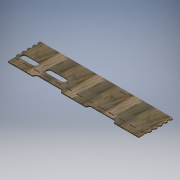
# Autodesk Inventor part: Dietro
Saved by Autodesk Inventor 2018.3 (Build 223284000, 284)
## iProperties
Created: 2019-03-05
Part Number: Dietro
Material: Generico
Document SubType Name: Modeling
Designer: AlfyPc
Density: 1 g/cm^3
Appearance: Legno alla deriva
Author: AlfyPc
Autodesk Inventor part; units mm, degrees
(part 1 of 5)
ref_plane "YZ Plane" through (0, 0, 0) normal (1, 0, 0) x (0, 1, 0)
ref_plane "XZ Plane" through (0, 0, 0) normal (0, 1, 0) x (-1, 0, 0)
ref_plane "XY Plane" through (0, 0, 0) normal (0, 0, 1) x (1, 0, 0)
sketch "Schizzo1" plane through (0, 0, 0) normal (0, 0, 1) x (1, 0, 0)
  line L0 (-15, -4) -> (-15, 0) construction
  line L1 (-34, 0) -> (-15, 0) construction
  line L2 (-53, 0) -> (-34, 0) construction
  line L3 (-72, 0) -> (-53, 0) construction
  line L4 (-91, 0) -> (-72, 0) construction
  line L5 (-110, 0) -> (-91, 0) construction
  line L6 (-129, 0) -> (-110, 0) construction
  line L7 (-148, 0) -> (-129, 0) construction
  line L8 (-167, 0) -> (-148, 0) construction
  line L9 (-186, 0) -> (-167, 0) construction
  line L10 (-205, 0) -> (-186, 0) construction
  line L11 (-224, 0) -> (-205, 0) construction
  line L12 (-243, 0) -> (-224, 0) construction
  line L13 (-262, 0) -> (-243, 0) construction
  line L14 (-281, 0) -> (-262, 0) construction
  line L15 (-300, 0) -> (-281, 0) construction
  line L16 (-319, 0) -> (-300, 0) construction
  line L17 (-338, 0) -> (-319, 0) construction
  line L18 (-357, 0) -> (-338, 0) construction
  line L19 (-376, 0) -> (-357, 0) construction
  line L20 (-395, 0) -> (-376, 0) construction
  line L21 (-414, 0) -> (-395, 0) construction
  line L22 (-433, 0) -> (-414, 0) construction
  line L23 (-452, 0) -> (-433, 0) construction
  line L24 (-471, 0) -> (-452, 0) construction
  line L25 (-471, -4) -> (-471, 0) construction
  line L26 (-452, -4) -> (-471, -4) construction
  line L27 (-452, 0) -> (-452, -4) construction
  line L28 (-15, -4) -> (-34, -4) construction
  line L29 (4, -4) -> (-15, -4) construction
  line L30 (4, 0) -> (4, -4) construction
  line L31 (-15, 0) -> (4, 0) construction
  line L32 (-34, 0) -> (-34, -4) construction
  line L33 (-53, -4) -> (-53, 0) construction
  line L34 (-34, -4) -> (-53, -4) construction
  line L35 (-72, 0) -> (-72, -4) construction
  line L36 (-53, -4) -> (-72, -4) construction
  line L37 (-91, -4) -> (-91, 0) construction
  line L38 (-72, -4) -> (-91, -4) construction
  line L39 (-110, 0) -> (-110, -4) construction
  line L40 (-91, -4) -> (-110, -4) construction
  line L41 (-129, -4) -> (-129, 0) construction
  line L42 (-110, -4) -> (-129, -4) construction
  line L43 (-148, 0) -> (-148, -4) construction
  line L44 (-129, -4) -> (-148, -4) construction
  line L45 (-167, -4) -> (-167, 0) construction
  line L46 (-148, -4) -> (-167, -4) construction
  line L47 (-186, 0) -> (-186, -4) construction
  line L48 (-167, -4) -> (-186, -4) construction
  line L49 (-205, -4) -> (-205, 0) construction
  line L50 (-186, -4) -> (-205, -4) construction
  line L51 (-224, 0) -> (-224, -4) construction
  line L52 (-205, -4) -> (-224, -4) construction
  line L53 (-243, -4) -> (-243, 0) construction
  line L54 (-224, -4) -> (-243, -4) construction
  line L55 (-262, 0) -> (-262, -4) construction
  line L56 (-243, -4) -> (-262, -4) construction
  line L57 (-281, -4) -> (-281, 0) construction
  line L58 (-262, -4) -> (-281, -4) construction
  line L59 (-300, 0) -> (-300, -4) construction
  line L60 (-281, -4) -> (-300, -4) construction
  line L61 (-319, -4) -> (-319, 0) construction
  line L62 (-300, -4) -> (-319, -4) construction
  line L63 (-338, 0) -> (-338, -4) construction
  line L64 (-319, -4) -> (-338, -4) construction
  line L65 (-357, -4) -> (-357, 0) construction
  line L66 (-338, -4) -> (-357, -4) construction
  line L67 (-376, 0) -> (-376, -4) construction
  line L68 (-357, -4) -> (-376, -4) construction
  line L69 (-395, -4) -> (-395, 0) construction
  line L70 (-376, -4) -> (-395, -4) construction
  line L71 (-414, 0) -> (-414, -4) construction
  line L72 (-395, -4) -> (-414, -4) construction
  line L73 (-433, -4) -> (-433, 0) construction
  line L74 (-414, -4) -> (-433, -4) construction
  line L75 (-433, -4) -> (-452, -4) construction
  line L76 (4, 95) -> (4, 0) construction
  line L77 (4, 0) -> (0, 0) construction
  line L78 (0, 0) -> (0, 95) construction
  line L79 (0, 95) -> (4, 95) construction
  line L80 (4, -4) -> (4, -24) construction
  line L81 (4, -24) -> (0, -24) construction
  line L82 (0, -24) -> (0, -4) construction
  line L83 (0, -4) -> (4, -4) construction
  line L84 (-381, -24) -> (-471, -24)
  line L85 (-471, -24) -> (-471, 95)
  line L86 (-471, 95) -> (4, 95)
  line L87 (4, 95) -> (4, -24)
  line L88 (-376, -19) -> (-376, -19)
  line L89 (-371, -14) -> (-286, -14)
  line L90 (-281, -19) -> (-281, -19)
  line L91 (-276, -24) -> (-191, -24)
  arc A0 (-381, -24) -> (-376, -19) centre (-381, -19) ccw
  arc A1 (-371, -14) -> (-376, -19) centre (-371, -19) ccw
  arc A2 (-281, -19) -> (-286, -14) centre (-286, -19) ccw
  arc A3 (-281, -19) -> (-276, -24) centre (-276, -19) ccw
  line L92 (-186, -19) -> (-186, -19)
  line L93 (-181, -14) -> (-96, -14)
  line L94 (-91, -19) -> (-91, -19)
  line L95 (-86, -24) -> (4, -24)
  arc A4 (-191, -24) -> (-186, -19) centre (-191, -19) ccw
  arc A5 (-181, -14) -> (-186, -19) centre (-181, -19) ccw
  arc A6 (-91, -19) -> (-96, -14) centre (-96, -19) ccw
  arc A7 (-91, -19) -> (-86, -24) centre (-86, -19) ccw
  line L96 (-15, -4) -> (4, -4) projected
  line L97 (4, 0) -> (4, -4) projected
  line L98 (4, 0) -> (-15, 0) projected
  line L99 (-15, 0) -> (-15, -4) projected
  line L100 (-53, -4) -> (-34, -4) projected
  line L101 (-34, 0) -> (-34, -4) projected
  line L102 (-53, 0) -> (-34, 0) projected
  line L103 (-53, 0) -> (-53, -4) projected
  line L104 (-91, -4) -> (-72, -4) projected
  line L105 (-72, 0) -> (-72, -4) projected
  line L106 (-91, 0) -> (-72, 0) projected
  line L107 (-91, 0) -> (-91, -4) projected
  line L108 (-129, -4) -> (-110, -4) projected
  line L109 (-110, 0) -> (-110, -4) projected
  line L110 (-129, 0) -> (-110, 0) projected
  line L111 (-129, 0) -> (-129, -4) projected
  line L112 (-167, -4) -> (-148, -4) projected
  line L113 (-148, 0) -> (-148, -4) projected
  line L114 (-167, 0) -> (-148, 0) projected
  line L115 (-167, 0) -> (-167, -4) projected
  line L116 (-205, -4) -> (-186, -4) projected
  line L117 (-186, 0) -> (-186, -4) projected
  line L118 (-205, 0) -> (-186, 0) projected
  line L119 (-205, 0) -> (-205, -4) projected
  line L120 (-243, -4) -> (-224, -4) projected
  line L121 (-224, 0) -> (-224, -4) projected
  line L122 (-243, 0) -> (-224, 0) projected
  line L123 (-243, 0) -> (-243, -4) projected
  line L124 (-281, -4) -> (-262, -4) projected
  line L125 (-262, 0) -> (-262, -4) projected
  line L126 (-281, 0) -> (-262, 0) projected
  line L127 (-281, 0) -> (-281, -4) projected
  line L128 (-319, -4) -> (-300, -4) projected
  line L129 (-300, 0) -> (-300, -4) projected
  line L130 (-319, 0) -> (-300, 0) projected
  line L131 (-319, 0) -> (-319, -4) projected
  line L132 (-357, -4) -> (-338, -4) projected
  line L133 (-338, 0) -> (-338, -4) projected
  line L134 (-357, 0) -> (-338, 0) projected
  line L135 (-357, 0) -> (-357, -4) projected
  line L136 (-395, -4) -> (-376, -4) projected
  line L137 (-376, 0) -> (-376, -4) projected
  line L138 (-395, 0) -> (-376, 0) projected
  line L139 (-395, 0) -> (-395, -4) projected
  line L140 (-433, -4) -> (-414, -4) projected
  line L141 (-414, 0) -> (-414, -4) projected
  line L142 (-433, 0) -> (-414, 0) projected
  line L143 (-433, 0) -> (-433, -4) projected
  line L144 (-471, -4) -> (-452, -4) projected
  line L145 (-452, 0) -> (-452, -4) projected
  line L146 (-471, 0) -> (-452, 0) projected
  line L147 (-471, 0) -> (-471, -4) projected
  line L148 (-361.5, 18) -> (-309.6633, 18) construction
  line L149 (-361.5, 8.6924) -> (-309.6633, 8.6924)
  line L150 (-309.6633, 27.3076) -> (-361.5, 27.3076)
  arc A8 (-361.5, 27.3076) -> (-361.5, 8.6924) centre (-361.5, 18) ccw
  arc A9 (-309.6633, 8.6924) -> (-309.6633, 27.3076) centre (-309.6633, 18) ccw
  line L151 (-451.5, 18) -> (-411.5, 18) construction
  line L152 (-451.5, 28) -> (-411.5, 28)
  line L153 (-411.5, 8) -> (-451.5, 8)
  arc A10 (-451.5, 28) -> (-451.5, 8) centre (-451.5, 18) ccw
  arc A11 (-411.5, 8) -> (-411.5, 28) centre (-411.5, 18) ccw
  point P0 (-376, -14)
  point P1 (-281, -14)
  point P2 (-281, -24)
  point P3 (-186, -24)
  point P4 (-186, -14)
  point P5 (-91, -14)
  point P6 (-335.5816, 18)
  point P7 (-431.5, 18)
  dimension "d2" = 95
  dimension "d3" = 90
  dimension "d4" = 95
  dimension "d5" = 5
  dimension "d6" = 90
  dimension "d7" = 95
  dimension "d8" = 5
  dimension "d22" = 40
  dimension "d23" = 18
  dimension "d24" = 20
  dimension "d25" = 50
  constraints: 208 end point, 56 horizontal, 31 vertical, 24 point on circle, 24 tangent, 17 point on line, 12 centre point, 6 equal radius, 6 perpendicular, 4 parallel, 2 midpoint, 57 other
  measures "d2" distance of point (-376, -14) point (-281, -14)
  measures "d3" angle of L88 L89
  measures "d4" distance of point (-281, -24) point (-186, -24)
  measures "d5" radius of A0
  measures "d6" distance of L84.start L84.end
  measures "d7" distance of point (-186, -14) point (-91, -14)
  measures "d8" radius of A4
  measures "d22" distance of L151.start L151.end
  measures "d23" distance between parallel lines of L22 L151
  measures "d24" distance between parallel lines of L153 L152
  measures "d25" distance of L151.end L148.start
extrude "Estrusione1" add sketch "Schizzo1" along normal blind 4 contours L84 L85 L144 L145 L146 L86 L87 L98 L99 L96 L95 A7 A6 L93 A5 A4 L91 A3 A2 L89 A1 A0
sketch "Schizzo2" plane through (0, 0, 4) normal (0, 0, 1) x (1, 0, 0)
  line L0 (0, -4) -> (0, -24) projected
  line L1 (0, -24) -> (4, -24) projected
  line L2 (4, -4) -> (4, -24) projected
  line L3 (0, -4) -> (4, -4) projected
  line L4 (0, -4) -> (0, -24) construction
  line L5 (4, -4) -> (4, -24) construction
  line L6 (-467, -4) -> (-471, -4) projected
  line L7 (-471, -24) -> (-471, -4) projected
  line L8 (-467, -24) -> (-471, -24) projected
  line L9 (-467, -24) -> (-467, -4) projected
  line L10 (-467, 0) -> (-467, 9.5) construction
  line L11 (-471, 0) -> (-471, 9.5) construction
  line L12 (4, 0) -> (4, 95) projected
  line L13 (0, 0) -> (4, 0)
  line L14 (4, 0) -> (4, 9.5)
  line L15 (4, 9.5) -> (0, 9.5)
  line L16 (0, 9.5) -> (0, 0)
  line L17 (-471, 95) -> (-471, 0) projected
  line L18 (-467, 0) -> (-471, 0)
  line L19 (-471, 0) -> (-471, 9.5)
  line L20 (-471, 9.5) -> (-467, 9.5)
  line L21 (-467, 9.5) -> (-467, 0)
  line L22 (0, 19) -> (0, 9.5)
  line L23 (0, 9.5) -> (4, 9.5)
  line L24 (4, 9.5) -> (4, 19)
  line L25 (4, 19) -> (0, 19)
  line L26 (-467, 19) -> (-467, 9.5)
  line L27 (-467, 9.5) -> (-471, 9.5)
  line L28 (-471, 9.5) -> (-471, 19)
  line L29 (-471, 19) -> (-467, 19)
  line L30 (0, 28.5) -> (0, 19)
  line L31 (0, 19) -> (4, 19)
  line L32 (4, 19) -> (4, 28.5)
  line L33 (4, 28.5) -> (0, 28.5)
  line L34 (-467, 28.5) -> (-467, 19)
  line L35 (-467, 19) -> (-471, 19)
  line L36 (-471, 19) -> (-471, 28.5)
  line L37 (-471, 28.5) -> (-467, 28.5)
  line L38 (0, 38) -> (0, 28.5)
  line L39 (0, 28.5) -> (4, 28.5)
  line L40 (4, 28.5) -> (4, 38)
  line L41 (4, 38) -> (0, 38)
  line L42 (-467, 38) -> (-467, 28.5)
  line L43 (-467, 28.5) -> (-471, 28.5)
  line L44 (-471, 28.5) -> (-471, 38)
  line L45 (-471, 38) -> (-467, 38)
  line L46 (0, 47.5) -> (0, 38)
  line L47 (0, 38) -> (4, 38)
  line L48 (4, 38) -> (4, 47.5)
  line L49 (4, 47.5) -> (0, 47.5)
  line L50 (-467, 47.5) -> (-467, 38)
  line L51 (-467, 38) -> (-471, 38)
  line L52 (-471, 38) -> (-471, 47.5)
  line L53 (-471, 47.5) -> (-467, 47.5)
  line L54 (0, 57) -> (0, 47.5)
  line L55 (0, 47.5) -> (4, 47.5)
  line L56 (4, 47.5) -> (4, 57)
  line L57 (4, 57) -> (0, 57)
  line L58 (-467, 57) -> (-467, 47.5)
  line L59 (-467, 47.5) -> (-471, 47.5)
  line L60 (-471, 47.5) -> (-471, 57)
  line L61 (-471, 57) -> (-467, 57)
  line L62 (0, 66.5) -> (0, 57)
  line L63 (0, 57) -> (4, 57)
  line L64 (4, 57) -> (4, 66.5)
  line L65 (4, 66.5) -> (0, 66.5)
  line L66 (-467, 66.5) -> (-467, 57)
  line L67 (-467, 57) -> (-471, 57)
  line L68 (-471, 57) -> (-471, 66.5)
  line L69 (-471, 66.5) -> (-467, 66.5)
  line L70 (0, 76) -> (0, 66.5)
  line L71 (0, 66.5) -> (4, 66.5)
  line L72 (4, 66.5) -> (4, 76)
  line L73 (4, 76) -> (0, 76)
  line L74 (-467, 76) -> (-467, 66.5)
  line L75 (-467, 66.5) -> (-471, 66.5)
  line L76 (-471, 66.5) -> (-471, 76)
  line L77 (-471, 76) -> (-467, 76)
  line L78 (0, 85.5) -> (0, 76)
  line L79 (0, 76) -> (4, 76)
  line L80 (4, 76) -> (4, 85.5)
  line L81 (4, 85.5) -> (0, 85.5)
  line L82 (-467, 85.5) -> (-467, 76)
  line L83 (-467, 76) -> (-471, 76)
  line L84 (-471, 76) -> (-471, 85.5)
  line L85 (-471, 85.5) -> (-467, 85.5)
  line L86 (0, 95) -> (0, 85.5)
  line L87 (0, 85.5) -> (4, 85.5)
  line L88 (4, 85.5) -> (4, 95)
  line L89 (4, 95) -> (0, 95)
  line L90 (-467, 95) -> (-467, 85.5)
  line L91 (-467, 85.5) -> (-471, 85.5)
  line L92 (-471, 85.5) -> (-471, 95)
  line L93 (-471, 95) -> (-467, 95)
  line L94 (0, -24) -> (4, -24) projected
  line L95 (0, -4) -> (4, -4) projected
  line L96 (-467, 9.5) -> (-471, 9.5) projected
  line L97 (-471, 0) -> (-467, 0) projected
  point P0 (4, 9.5)
  point P1 (-471, 9.5)
  point P2 (4, 19)
  point P3 (-471, 19)
  point P4 (4, 28.5)
  point P5 (-471, 28.5)
  point P6 (4, 38)
  point P7 (-471, 38)
  point P8 (4, 47.5)
  point P9 (-471, 47.5)
  point P10 (4, 57)
  point P11 (-471, 57)
  point P12 (4, 66.5)
  point P13 (-471, 66.5)
  point P14 (4, 76)
  point P15 (-471, 76)
  point P16 (4, 85.5)
  point P17 (-471, 85.5)
  point P18 (-471, 9.5)
  dimension "d11" = 9.5
  dimension "d12" = 9.5
  dimension "d15" = 9.5
  constraints: 160 end point, 4 parallel, 2 horizontal, 2 perpendicular, 2 point on line, 1 vertical, 162 other
  measures "d11" distance of L14.end L13.end
  measures "d12" distance of L18.end L11.end
  measures "d15" distance of L13.start L22.end
extrude "Estrusione2" cut sketch "Schizzo2" against normal blind 4 contours L3 L2 L1 L0 | L9 L8 L7 L6 | L13 L16 L15 L12 | L25 L30 L33 L12 | L41 L46 L49 L12 | L57 L62 L65 L12 | L73 L78 L81 L12 | L85 L82 L77 L17 | L69 L66 L61 L17 | L53 L50 L45 L17 | L37 L34 L29 L17 | L20 L21 L18 L17
sketch "Schizzo3" plane through (0, 0, 4) normal (0, 0, 1) x (1, 0, 0)
  line L0 (-444.15, 0) -> (-440.85, 0) projected
  line L1 (-292.15, 0) -> (-288.85, 0) projected
  line L2 (-26.15, 0) -> (-22.85, 0) projected
  line L3 (-290.5, 0) -> (-290.5, 13) construction
  circle A0 centre (-290.5, 13) radius 1.65
  line L4 (0, -24) -> (0, -4) projected
  line L5 (0, -4) -> (-15, -4) projected
  line L6 (-15, -4) -> (-15, 0) projected
  line L7 (-15, 0) -> (0, 0) projected
  line L8 (0, 0) -> (0, 9.5) projected
  line L9 (0, 9.5) -> (4, 9.5) projected
  line L10 (4, 9.5) -> (4, 19) projected
  line L11 (4, 19) -> (0, 19) projected
  line L12 (0, 19) -> (0, 28.5) projected
  line L13 (0, 28.5) -> (4, 28.5) projected
  line L14 (4, 28.5) -> (4, 38) projected
  line L15 (4, 38) -> (0, 38) projected
  line L16 (0, 38) -> (0, 47.5) projected
  line L17 (0, 47.5) -> (4, 47.5) projected
  line L18 (4, 47.5) -> (4, 57) projected
  line L19 (4, 57) -> (0, 57) projected
  line L20 (0, 57) -> (0, 66.5) projected
  line L21 (0, 66.5) -> (4, 66.5) projected
  line L22 (4, 66.5) -> (4, 76) projected
  line L23 (4, 76) -> (0, 76) projected
  line L24 (0, 76) -> (0, 85.5) projected
  line L25 (0, 85.5) -> (4, 85.5) projected
  line L26 (4, 85.5) -> (4, 95) projected
  line L27 (4, 95) -> (-471, 95) projected
  line L28 (-471, 95) -> (-471, 85.5) projected
  line L29 (-471, 85.5) -> (-467, 85.5) projected
  line L30 (-467, 85.5) -> (-467, 76) projected
  line L31 (-467, 76) -> (-471, 76) projected
  line L32 (-471, 76) -> (-471, 66.5) projected
  line L33 (-471, 66.5) -> (-467, 66.5) projected
  line L34 (-467, 66.5) -> (-467, 57) projected
  line L35 (-467, 57) -> (-471, 57) projected
  line L36 (-471, 57) -> (-471, 47.5) projected
  line L37 (-471, 47.5) -> (-467, 47.5) projected
  line L38 (-467, 47.5) -> (-467, 38) projected
  line L39 (-467, 38) -> (-471, 38) projected
  line L40 (-471, 38) -> (-471, 28.5) projected
  line L41 (-471, 28.5) -> (-467, 28.5) projected
  line L42 (-467, 28.5) -> (-467, 19) projected
  line L43 (-467, 19) -> (-471, 19) projected
  line L44 (-471, 19) -> (-471, 9.5) projected
  line L45 (-471, 9.5) -> (-467, 9.5) projected
  line L46 (-467, 9.5) -> (-467, 0) projected
  line L47 (-467, 0) -> (-452, 0) projected
  line L48 (-452, 0) -> (-452, -4) projected
  line L49 (-452, -4) -> (-467, -4) projected
  line L50 (-467, -4) -> (-467, -24) projected
  line L51 (-467, -24) -> (-381, -24) projected
  arc A1 (-381, -24) -> (-376, -19) centre (-381, -19) ccw projected
  arc A2 (-371, -14) -> (-376, -19) centre (-371, -19) ccw projected
  line L52 (-371, -14) -> (-286, -14) projected
  arc A3 (-281, -19) -> (-286, -14) centre (-286, -19) ccw projected
  arc A4 (-281, -19) -> (-276, -24) centre (-276, -19) ccw projected
  line L53 (-276, -24) -> (-191, -24) projected
  arc A5 (-191, -24) -> (-186, -19) centre (-191, -19) ccw projected
  arc A6 (-181, -14) -> (-186, -19) centre (-181, -19) ccw projected
  line L54 (-181, -14) -> (-96, -14) projected
  arc A7 (-91, -19) -> (-96, -14) centre (-96, -19) ccw projected
  arc A8 (-91, -19) -> (-86, -24) centre (-86, -19) ccw projected
  line L55 (-86, -24) -> (0, -24) projected
  arc A9 (-361.5, 27.3076) -> (-361.5, 8.6924) centre (-361.5, 18) ccw projected
  line L56 (-361.5, 27.3076) -> (-309.6633, 27.3076) projected
  arc A10 (-309.6633, 8.6924) -> (-309.6633, 27.3076) centre (-309.6633, 18) ccw projected
  line L57 (-309.6633, 8.6924) -> (-361.5, 8.6924) projected
  arc A11 (-411.5, 8) -> (-411.5, 28) centre (-411.5, 18) ccw projected
  line L58 (-411.5, 8) -> (-451.5, 8) projected
  arc A12 (-451.5, 28) -> (-451.5, 8) centre (-451.5, 18) ccw projected
  line L59 (-451.5, 28) -> (-411.5, 28) projected
  line L60 (-34, -4) -> (-53, -4) projected
  line L61 (-53, -4) -> (-53, 0) projected
  line L62 (-53, 0) -> (-34, 0) projected
  line L63 (-34, 0) -> (-34, -4) projected
  line L64 (-72, -4) -> (-91, -4) projected
  line L65 (-91, -4) -> (-91, 0) projected
  line L66 (-91, 0) -> (-72, 0) projected
  line L67 (-72, 0) -> (-72, -4) projected
  line L68 (-110, -4) -> (-129, -4) projected
  line L69 (-129, -4) -> (-129, 0) projected
  line L70 (-129, 0) -> (-110, 0) projected
  line L71 (-110, 0) -> (-110, -4) projected
  line L72 (-148, -4) -> (-167, -4) projected
  line L73 (-167, -4) -> (-167, 0) projected
  line L74 (-167, 0) -> (-148, 0) projected
  line L75 (-148, 0) -> (-148, -4) projected
  line L76 (-186, -4) -> (-205, -4) projected
  line L77 (-205, -4) -> (-205, 0) projected
  line L78 (-205, 0) -> (-186, 0) projected
  line L79 (-186, 0) -> (-186, -4) projected
  line L80 (-224, -4) -> (-243, -4) projected
  line L81 (-243, -4) -> (-243, 0) projected
  line L82 (-243, 0) -> (-224, 0) projected
  line L83 (-224, 0) -> (-224, -4) projected
  line L84 (-262, -4) -> (-281, -4) projected
  line L85 (-281, -4) -> (-281, 0) projected
  line L86 (-281, 0) -> (-262, 0) projected
  line L87 (-262, 0) -> (-262, -4) projected
  line L88 (-300, -4) -> (-319, -4) projected
  line L89 (-319, -4) -> (-319, 0) projected
  line L90 (-319, 0) -> (-300, 0) projected
  line L91 (-300, 0) -> (-300, -4) projected
  line L92 (-338, -4) -> (-357, -4) projected
  line L93 (-357, -4) -> (-357, 0) projected
  line L94 (-357, 0) -> (-338, 0) projected
  line L95 (-338, 0) -> (-338, -4) projected
  line L96 (-376, -4) -> (-395, -4) projected
  line L97 (-395, -4) -> (-395, 0) projected
  line L98 (-395, 0) -> (-376, 0) projected
  line L99 (-376, 0) -> (-376, -4) projected
  line L100 (-414, -4) -> (-433, -4) projected
  line L101 (-433, -4) -> (-433, 0) projected
  line L102 (-433, 0) -> (-414, 0) projected
  line L103 (-414, 0) -> (-414, -4) projected
  line L104 (-467, 85.5) -> (-467, 76) construction
  line L105 (-467, 80.75) -> (-454, 80.75) construction
  line L106 (0, 85.5) -> (0, 76) construction
  line L107 (0, 80.75) -> (-13, 80.75) construction
  line L108 (0, -4) -> (0, -24) construction
  line L109 (0, -14) -> (-13, -14) construction
  line L110 (-467, -24) -> (-467, -4) construction
  line L111 (-467, -14) -> (-454, -14) construction
  circle A13 centre (-454, -14) radius 1.65
  circle A14 centre (-454, 80.75) radius 1.65
  circle A15 centre (-13, 80.75) radius 1.65
  circle A16 centre (-13, -14) radius 1.65
  dimension "d28" = 13
  dimension "d30" = 3.3
  dimension "d38" = 13
  dimension "d39" = 13
  dimension "d40" = 13
  dimension "d41" = 13
  dimension "d42" = 3.3
  dimension "d43" = 3.3
  dimension "d44" = 3.3
  dimension "d45" = 3.3
  constraints: 10 end point, 5 centre point, 5 coincident, 5 midpoint, 4 horizontal, 1 vertical
  measures "d28" distance of L3.start L3.end
  measures "d30" diameter of A0
  measures "d38" distance of L105.start L105.end
  measures "d39" distance of L107.start L107.end
  measures "d40" distance of L109.start L109.end
  measures "d41" distance of L111.start L111.end
  measures "d42" diameter of A13
  measures "d43" diameter of A14
  measures "d44" diameter of A15
  measures "d45" diameter of A16
extrude "Estrusione3" cut sketch "Schizzo3" against normal blind 4 contours A0 | A13 | A14 | A15 | A16
sketch "Schizzo5" plane through (0, 0, 0) normal (0, 0, -1) x (-1, 0, 0)
  line L0 (154, 85) -> (174, 85)
  line L1 (174, 85) -> (174, 82)
  line L2 (174, 82) -> (154, 82)
  line L3 (154, 82) -> (154, 85)
  line L4 (174, 51) -> (154, 51)
  line L5 (154, 51) -> (154, 54)
  line L6 (154, 54) -> (174, 54)
  line L7 (174, 54) -> (174, 51)
  point P0 (0, 0)
  dimension "d35" = 3
  constraints: 16 end point, 4 parallel, 2 horizontal, 2 perpendicular
  measures "d35" distance of L4.end L5.end
extrude "Estrusione4" cut sketch "Schizzo5" against normal blind 11.25
sketch "Schizzo6" plane through (0, 0, 4) normal (0, 0, 1) x (1, 0, 0)
  line L0 (-271.9016, 69.693) -> (-208.9989, 69.693) construction
  line L1 (-208.9989, 69.693) -> (-208.9989, 48.9432) construction
  line L2 (-208.9989, 48.9432) -> (-271.9016, 48.9432) construction
  line L3 (-271.9016, 48.9432) -> (-271.9016, 69.693) construction
  line L4 (-445.1797, 85.8425) -> (-407.7445, 85.8425)
  line L5 (-407.7445, 85.8425) -> (-407.7445, 37)
  line L6 (-407.7445, 37) -> (-445.1797, 37)
  line L7 (-445.1797, 37) -> (-445.1797, 85.8425)
  line L8 (-312.8687, 85.8425) -> (-290, 85.8425)
  line L9 (-290, 85.8425) -> (-290, 38)
  line L10 (-290, 38) -> (-312.8687, 38)
  line L11 (-312.8687, 38) -> (-312.8687, 85.8425)
  line L12 (-399.6431, 87.7398) -> (-345.391, 87.7398) construction
  line L13 (-345.391, 87.7398) -> (-345.391, 36.9673) construction
  line L14 (-345.391, 36.9673) -> (-399.6431, 36.9673) construction
  line L15 (-399.6431, 36.9673) -> (-399.6431, 87.7398) construction
  spline S0 degree 2 poles (-396.4657, 86.079) (-396.4657, 85.615) (-396.8562, 84.902) (-397.5777, 84.5144) (-398.0502, 84.5144) knots 0 0 0 1 2 3 3 3
  line L16 (-398.0502, 84.5144) -> (-399.3432, 84.5144)
  line L17 (-399.3432, 84.5144) -> (-399.3432, 87.5644)
  line L18 (-399.3432, 87.5644) -> (-398.0785, 87.5644)
  spline S1 degree 2 poles (-398.0785, 87.5644) (-396.4657, 87.5644) (-396.4657, 86.079) knots 0 0 0 1 1 1
  spline S2 degree 2 poles (-397.4419, 86.0705) (-397.4419, 86.2912) (-397.6229, 86.6505) (-397.9596, 86.8457) (-398.186, 86.8457) knots 0 0 0 1 2 3 3 3
  line L19 (-398.186, 86.8457) -> (-398.4236, 86.8457)
  line L20 (-398.4236, 86.8457) -> (-398.4236, 85.233)
  line L21 (-398.4236, 85.233) -> (-398.1662, 85.233)
  spline S3 degree 2 poles (-398.1662, 85.233) (-397.8351, 85.233) (-397.4419, 85.6857) (-397.4419, 86.0705) knots 0 0 0 1 2 2 2
  spline S4 degree 2 poles (-395.3368, 85.3462) (-395.3142, 85.2047) (-395.0369, 85.0463) (-394.8106, 85.0463) knots 0 0 0 1 2 2 2
  spline S5 degree 2 poles (-394.8106, 85.0463) (-394.4937, 85.0463) (-394.2108, 85.1679) knots 0 0 0 1 1 1
  line L22 (-394.2108, 85.1679) -> (-394.2108, 84.5936)
  spline S6 degree 2 poles (-394.2108, 84.5936) (-394.539, 84.4606) (-395.0115, 84.4606) knots 0 0 0 1 1 1
  spline S7 degree 2 poles (-395.0115, 84.4606) (-395.5802, 84.4606) (-396.2139, 85.0435) (-396.2139, 85.5556) knots 0 0 0 1 2 2 2
  spline S8 degree 2 poles (-396.2139, 85.5556) (-396.2139, 85.9064) (-395.9367, 86.4411) (-395.3906, 86.7467) (-395.0596, 86.7467) knots 0 0 0 1 2 3 3 3
  spline S9 degree 2 poles (-395.0596, 86.7467) (-394.7229, 86.7467) (-394.2419, 86.4836) (-393.9929, 86.0054) (-393.9929, 85.6857) knots 0 0 0 1 2 3 3 3
  line L23 (-393.9929, 85.6857) -> (-393.9929, 85.3462)
  line L24 (-393.9929, 85.3462) -> (-395.3368, 85.3462)
  spline S10 degree 2 poles (-394.7936, 85.8215) (-394.7936, 86.1978) (-395.0624, 86.1978) knots 0 0 0 1 1 1
  spline S11 degree 2 poles (-395.0624, 86.1978) (-395.1756, 86.1978) (-395.3284, 85.9913) (-395.3425, 85.8215) knots 0 0 0 1 2 2 2
  line L25 (-395.3425, 85.8215) -> (-394.7936, 85.8215)
  line L26 (-392.0945, 84.5144) -> (-393.1696, 84.5144)
  line L27 (-393.1696, 84.5144) -> (-393.8967, 86.6929)
  line L28 (-393.8967, 86.6929) -> (-392.9517, 86.6929)
  line L29 (-392.9517, 86.6929) -> (-392.6858, 85.5046)
  spline S12 degree 2 poles (-392.6858, 85.5046) (-392.6235, 85.216) (-392.615, 85.0718) knots 0 0 0 1 1 1
  line L30 (-392.615, 85.0718) -> (-392.6037, 85.0718)
  spline S13 degree 2 poles (-392.6037, 85.0718) (-392.5981, 85.1142) (-392.5839, 85.2047) (-392.2755, 86.6929) knots 0 0 0 1 2 2 2
  line L31 (-392.2755, 86.6929) -> (-391.3362, 86.6929)
  line L32 (-391.3362, 86.6929) -> (-392.0945, 84.5144)
  spline S14 degree 2 poles (-390.3375, 85.3462) (-390.3148, 85.2047) (-390.0375, 85.0463) (-389.8112, 85.0463) knots 0 0 0 1 2 2 2
  spline S15 degree 2 poles (-389.8112, 85.0463) (-389.4943, 85.0463) (-389.2114, 85.1679) knots 0 0 0 1 1 1
  line L33 (-389.2114, 85.1679) -> (-389.2114, 84.5936)
  spline S16 degree 2 poles (-389.2114, 84.5936) (-389.5396, 84.4606) (-390.0121, 84.4606) knots 0 0 0 1 1 1
  spline S17 degree 2 poles (-390.0121, 84.4606) (-390.5808, 84.4606) (-391.2145, 85.0435) (-391.2145, 85.5556) knots 0 0 0 1 2 2 2
  spline S18 degree 2 poles (-391.2145, 85.5556) (-391.2145, 85.9064) (-390.9373, 86.4411) (-390.3912, 86.7467) (-390.0602, 86.7467) knots 0 0 0 1 2 3 3 3
  spline S19 degree 2 poles (-390.0602, 86.7467) (-389.7235, 86.7467) (-389.2425, 86.4836) (-388.9935, 86.0054) (-388.9935, 85.6857) knots 0 0 0 1 2 3 3 3
  line L34 (-388.9935, 85.6857) -> (-388.9935, 85.3462)
  line L35 (-388.9935, 85.3462) -> (-390.3375, 85.3462)
  spline S20 degree 2 poles (-389.7942, 85.8215) (-389.7942, 86.1978) (-390.063, 86.1978) knots 0 0 0 1 1 1
  spline S21 degree 2 poles (-390.063, 86.1978) (-390.1762, 86.1978) (-390.329, 85.9913) (-390.3431, 85.8215) knots 0 0 0 1 2 2 2
  line L36 (-390.3431, 85.8215) -> (-389.7942, 85.8215)
  line L37 (-388.6795, 84.5144) -> (-388.6795, 87.7398)
  line L38 (-388.6795, 87.7398) -> (-387.7741, 87.7398)
  line L39 (-387.7741, 87.7398) -> (-387.7741, 84.5144)
  line L40 (-387.7741, 84.5144) -> (-388.6795, 84.5144)
  spline S22 degree 2 poles (-384.9165, 85.6433) (-384.9165, 85.0916) (-385.5814, 84.4606) (-386.1784, 84.4606) knots 0 0 0 1 2 2 2
  spline S23 degree 2 poles (-386.1784, 84.4606) (-386.7725, 84.4606) (-387.4346, 85.0746) (-387.4346, 85.6178) knots 0 0 0 1 2 2 2
  spline S24 degree 2 poles (-387.4346, 85.6178) (-387.4346, 85.963) (-387.1234, 86.4751) (-386.549, 86.7467) (-386.1755, 86.7467) knots 0 0 0 1 2 3 3 3
  spline S25 degree 2 poles (-386.1755, 86.7467) (-385.7879, 86.7467) (-385.2192, 86.4609) (-384.9165, 85.9545) (-384.9165, 85.6433) knots 0 0 0 1 2 3 3 3
  spline S26 degree 2 poles (-385.836, 85.6376) (-385.836, 86.0818) (-386.1755, 86.0818) knots 0 0 0 1 1 1
  spline S27 degree 2 poles (-386.1755, 86.0818) (-386.515, 86.0818) (-386.515, 85.6178) knots 0 0 0 1 1 1
  spline S28 degree 2 poles (-386.515, 85.6178) (-386.515, 85.1255) (-386.1699, 85.1255) knots 0 0 0 1 1 1
  spline S29 degree 2 poles (-386.1699, 85.1255) (-385.836, 85.1255) (-385.836, 85.6376) knots 0 0 0 1 1 1
  spline S30 degree 2 poles (-382.1211, 85.6687) (-382.1211, 85.3122) (-382.3644, 84.7634) (-382.8058, 84.4606) (-383.0831, 84.4606) knots 0 0 0 1 2 3 3 3
  spline S31 degree 2 poles (-383.0831, 84.4606) (-383.465, 84.4606) (-383.6631, 84.7407) knots 0 0 0 1 1 1
  line L41 (-383.6631, 84.7407) -> (-383.6716, 84.7407)
  line L42 (-383.6716, 84.7407) -> (-383.6716, 83.5128)
  line L43 (-383.6716, 83.5128) -> (-384.577, 83.5128)
  line L44 (-384.577, 83.5128) -> (-384.577, 86.6929)
  line L45 (-384.577, 86.6929) -> (-383.6716, 86.6929)
  line L46 (-383.6716, 86.6929) -> (-383.6716, 86.3959)
  line L47 (-383.6716, 86.3959) -> (-383.6631, 86.3959)
  spline S32 degree 2 poles (-383.6631, 86.3959) (-383.5556, 86.56) (-383.2104, 86.7467) (-382.9897, 86.7467) knots 0 0 0 1 2 2 2
  spline S33 degree 2 poles (-382.9897, 86.7467) (-382.571, 86.7467) (-382.1211, 86.1837) (-382.1211, 85.6687) knots 0 0 0 1 2 2 2
  spline S34 degree 2 poles (-383.0407, 85.6433) (-383.0407, 85.847) (-383.1991, 86.0818) (-383.366, 86.0818) knots 0 0 0 1 2 2 2
  spline S35 degree 2 poles (-383.366, 86.0818) (-383.5103, 86.0818) (-383.6886, 85.8357) (-383.6886, 85.6206) knots 0 0 0 1 2 2 2
  line L48 (-383.6886, 85.6206) -> (-383.6886, 85.5782)
  spline S36 degree 2 poles (-383.6886, 85.5782) (-383.6886, 85.3717) (-383.5358, 85.1255) (-383.383, 85.1255) knots 0 0 0 1 2 2 2
  spline S37 degree 2 poles (-383.383, 85.1255) (-383.2189, 85.1255) (-383.0407, 85.3943) (-383.0407, 85.6433) knots 0 0 0 1 2 2 2
  spline S38 degree 2 poles (-380.9979, 85.3462) (-380.9753, 85.2047) (-380.698, 85.0463) (-380.4716, 85.0463) knots 0 0 0 1 2 2 2
  spline S39 degree 2 poles (-380.4716, 85.0463) (-380.1548, 85.0463) (-379.8718, 85.1679) knots 0 0 0 1 1 1
  line L49 (-379.8718, 85.1679) -> (-379.8718, 84.5936)
  spline S40 degree 2 poles (-379.8718, 84.5936) (-380.2, 84.4606) (-380.6725, 84.4606) knots 0 0 0 1 1 1
  spline S41 degree 2 poles (-380.6725, 84.4606) (-381.2412, 84.4606) (-381.875, 85.0435) (-381.875, 85.5556) knots 0 0 0 1 2 2 2
  spline S42 degree 2 poles (-381.875, 85.5556) (-381.875, 85.9064) (-381.5977, 86.4411) (-381.0516, 86.7467) (-380.7206, 86.7467) knots 0 0 0 1 2 3 3 3
  spline S43 degree 2 poles (-380.7206, 86.7467) (-380.3839, 86.7467) (-379.9029, 86.4836) (-379.654, 86.0054) (-379.654, 85.6857) knots 0 0 0 1 2 3 3 3
  line L50 (-379.654, 85.6857) -> (-379.654, 85.3462)
  line L51 (-379.654, 85.3462) -> (-380.9979, 85.3462)
  spline S44 degree 2 poles (-380.4547, 85.8215) (-380.4547, 86.1978) (-380.7234, 86.1978) knots 0 0 0 1 1 1
  spline S45 degree 2 poles (-380.7234, 86.1978) (-380.8366, 86.1978) (-380.9894, 85.9913) (-381.0035, 85.8215) knots 0 0 0 1 2 2 2
  line L52 (-381.0035, 85.8215) -> (-380.4547, 85.8215)
  line L53 (-377.8856, 84.5144) -> (-377.8856, 84.769)
  line L54 (-377.8856, 84.769) -> (-377.8941, 84.769)
  spline S46 degree 2 poles (-377.8941, 84.769) (-378.0016, 84.6247) (-378.3525, 84.4606) (-378.5222, 84.4606) knots 0 0 0 1 2 2 2
  spline S47 degree 2 poles (-378.5222, 84.4606) (-378.7995, 84.4606) (-379.2267, 84.7351) (-379.4361, 85.2302) (-379.4361, 85.5641) knots 0 0 0 1 2 3 3 3
  spline S48 degree 2 poles (-379.4361, 85.5641) (-379.4361, 85.9121) (-379.1843, 86.4496) (-378.7288, 86.7467) (-378.4458, 86.7467) knots 0 0 0 1 2 3 3 3
  spline S49 degree 2 poles (-378.4458, 86.7467) (-378.3129, 86.7467) (-378.0865, 86.6703) (-377.9168, 86.5402) (-377.8941, 86.4751) knots 0 0 0 1 2 3 3 3
  line L55 (-377.8941, 86.4751) -> (-377.8856, 86.4751)
  line L56 (-377.8856, 86.4751) -> (-377.8856, 87.7398)
  line L57 (-377.8856, 87.7398) -> (-376.9803, 87.7398)
  line L58 (-376.9803, 87.7398) -> (-376.9803, 84.5144)
  line L59 (-376.9803, 84.5144) -> (-377.8856, 84.5144)
  spline S50 degree 2 poles (-377.8658, 85.6687) (-377.8658, 85.864) (-378.0384, 86.0818) (-378.1856, 86.0818) knots 0 0 0 1 2 2 2
  spline S51 degree 2 poles (-378.1856, 86.0818) (-378.3327, 86.0818) (-378.5166, 85.813) (-378.5166, 85.5867) knots 0 0 0 1 2 2 2
  spline S52 degree 2 poles (-378.5166, 85.5867) (-378.5166, 85.1255) (-378.1969, 85.1255) knots 0 0 0 1 1 1
  spline S53 degree 2 poles (-378.1969, 85.1255) (-378.0469, 85.1255) (-377.8658, 85.3745) (-377.8658, 85.6122) knots 0 0 0 1 2 2 2
  line L60 (-377.8658, 85.6122) -> (-377.8658, 85.6687)
  spline S54 degree 2 poles (-372.8749, 85.6687) (-372.8749, 85.3122) (-373.1098, 84.7605) (-373.5455, 84.4606) (-373.8199, 84.4606) knots 0 0 0 1 2 3 3 3
  spline S55 degree 2 poles (-373.8199, 84.4606) (-374.0293, 84.4606) (-374.3292, 84.6162) (-374.4169, 84.7407) knots 0 0 0 1 2 2 2
  line L61 (-374.4169, 84.7407) -> (-374.4254, 84.7407)
  line L62 (-374.4254, 84.7407) -> (-374.4254, 84.5144)
  line L63 (-374.4254, 84.5144) -> (-375.3308, 84.5144)
  line L64 (-375.3308, 84.5144) -> (-375.3308, 87.7398)
  line L65 (-375.3308, 87.7398) -> (-374.4254, 87.7398)
  line L66 (-374.4254, 87.7398) -> (-374.4254, 86.3987)
  line L67 (-374.4254, 86.3987) -> (-374.4169, 86.3987)
  spline S56 degree 2 poles (-374.4169, 86.3987) (-374.3094, 86.56) (-373.9472, 86.7467) (-373.7266, 86.7467) knots 0 0 0 1 2 2 2
  spline S57 degree 2 poles (-373.7266, 86.7467) (-373.3163, 86.7467) (-372.8749, 86.1978) (-372.8749, 85.6687) knots 0 0 0 1 2 2 2
  spline S58 degree 2 poles (-373.7945, 85.6433) (-373.7945, 85.8611) (-373.9614, 86.0818) (-374.1198, 86.0818) knots 0 0 0 1 2 2 2
  spline S59 degree 2 poles (-374.1198, 86.0818) (-374.2585, 86.0818) (-374.4424, 85.8498) (-374.4424, 85.6659) knots 0 0 0 1 2 2 2
  line L68 (-374.4424, 85.6659) -> (-374.4424, 85.5329)
  spline S60 degree 2 poles (-374.4424, 85.5329) (-374.4424, 85.3462) (-374.2754, 85.1255) (-374.1368, 85.1255) knots 0 0 0 1 2 2 2
  spline S61 degree 2 poles (-374.1368, 85.1255) (-373.9727, 85.1255) (-373.7945, 85.3943) (-373.7945, 85.6433) knots 0 0 0 1 2 2 2
  spline S62 degree 2 poles (-372.111, 83.4902) (-372.2383, 83.4902) (-372.5298, 83.5354) (-372.6458, 83.5779) knots 0 0 0 1 2 2 2
  line L69 (-372.6458, 83.5779) -> (-372.6458, 84.2597)
  spline S63 degree 2 poles (-372.6458, 84.2597) (-372.592, 84.2201) (-372.3826, 84.1522) (-372.2893, 84.1522) knots 0 0 0 1 2 2 2
  spline S64 degree 2 poles (-372.2893, 84.1522) (-372.0346, 84.1522) (-371.9526, 84.3531) knots 0 0 0 1 1 1
  line L70 (-371.9526, 84.3531) -> (-371.8818, 84.5229)
  line L71 (-371.8818, 84.5229) -> (-372.7929, 86.6929)
  line L72 (-372.7929, 86.6929) -> (-371.7913, 86.6929)
  line L73 (-371.7913, 86.6929) -> (-371.5282, 85.6433)
  spline S65 degree 2 poles (-371.5282, 85.6433) (-371.4518, 85.349) (-371.4433, 85.2472) knots 0 0 0 1 1 1
  line L74 (-371.4433, 85.2472) -> (-371.4348, 85.2472)
  spline S66 degree 2 poles (-371.4348, 85.2472) (-371.4291, 85.2953) (-371.4065, 85.4084) (-371.0868, 86.6929) knots 0 0 0 1 2 2 2
  line L75 (-371.0868, 86.6929) -> (-370.2069, 86.6929)
  line L76 (-370.2069, 86.6929) -> (-371.0076, 84.4521)
  spline S67 degree 2 poles (-371.0076, 84.4521) (-371.1887, 83.9372) (-371.7234, 83.4902) (-372.111, 83.4902) knots 0 0 0 1 2 2 2
  spline S68 degree 2 poles (-369.0469, 84.8935) (-369.0469, 84.6983) (-369.3185, 84.4606) (-369.559, 84.4606) knots 0 0 0 1 2 2 2
  spline S69 degree 2 poles (-369.559, 84.4606) (-369.7797, 84.4606) (-370.0569, 84.7096) (-370.0569, 84.8935) knots 0 0 0 1 2 2 2
  spline S70 degree 2 poles (-370.0569, 84.8935) (-370.0569, 85.0802) (-369.7825, 85.3122) (-369.5505, 85.3122) knots 0 0 0 1 2 2 2
  spline S71 degree 2 poles (-369.5505, 85.3122) (-369.3241, 85.3122) (-369.0469, 85.0802) (-369.0469, 84.8935) knots 0 0 0 1 2 2 2
  spline S72 degree 2 poles (-369.0469, 86.2742) (-369.0469, 86.079) (-369.3213, 85.8442) (-369.559, 85.8442) knots 0 0 0 1 2 2 2
  spline S73 degree 2 poles (-369.559, 85.8442) (-369.7768, 85.8442) (-370.0569, 86.0903) (-370.0569, 86.2742) knots 0 0 0 1 2 2 2
  spline S74 degree 2 poles (-370.0569, 86.2742) (-370.0569, 86.4609) (-369.7825, 86.6929) (-369.5505, 86.6929) knots 0 0 0 1 2 2 2
  spline S75 degree 2 poles (-369.5505, 86.6929) (-369.3241, 86.6929) (-369.0469, 86.4609) (-369.0469, 86.2742) knots 0 0 0 1 2 2 2
  spline S76 degree 2 poles (-398.07, 79.6161) (-398.07, 79.452) (-398.2397, 79.1606) (-398.5311, 78.9936) (-398.6924, 78.9936) knots 0 0 0 1 2 3 3 3
  spline S77 degree 2 poles (-398.6924, 78.9936) (-398.9442, 78.9936) (-399.3064, 79.3558) (-399.3064, 79.6161) knots 0 0 0 1 2 2 2
  spline S78 degree 2 poles (-399.3064, 79.6161) (-399.3064, 79.8679) (-398.9499, 80.23) (-398.6924, 80.23) knots 0 0 0 1 2 2 2
  spline S79 degree 2 poles (-398.6924, 80.23) (-398.4293, 80.23) (-398.07, 79.8622) (-398.07, 79.6161) knots 0 0 0 1 2 2 2
  line L77 (-388.2805, 78.5777) -> (-388.4135, 79.1379)
  line L78 (-388.4135, 79.1379) -> (-389.3246, 79.1379)
  line L79 (-389.3246, 79.1379) -> (-389.4689, 78.5777)
  line L80 (-389.4689, 78.5777) -> (-390.4619, 78.5777)
  line L81 (-390.4619, 78.5777) -> (-389.4123, 81.6277)
  line L82 (-389.4123, 81.6277) -> (-388.2721, 81.6277)
  line L83 (-388.2721, 81.6277) -> (-387.2818, 78.5777)
  line L84 (-387.2818, 78.5777) -> (-388.2805, 78.5777)
  line L85 (-388.8577, 80.9628) -> (-388.8775, 80.9628)
  spline S80 degree 2 poles (-388.8775, 80.9628) (-388.8832, 80.9119) (-388.9341, 80.6771) (-389.1661, 79.7915) knots 0 0 0 1 2 2 2
  line L86 (-389.1661, 79.7915) -> (-388.5833, 79.7915)
  line L87 (-388.5833, 79.7915) -> (-388.7955, 80.6205)
  spline S81 degree 2 poles (-388.7955, 80.6205) (-388.8407, 80.8044) (-388.8577, 80.9628) knots 0 0 0 1 1 1
  line L88 (-387.0074, 78.5777) -> (-387.0074, 81.8031)
  line L89 (-387.0074, 81.8031) -> (-386.102, 81.8031)
  line L90 (-386.102, 81.8031) -> (-386.102, 78.5777)
  line L91 (-386.102, 78.5777) -> (-387.0074, 78.5777)
  spline S82 degree 2 poles (-383.9885, 81.1439) (-384.1299, 81.192) (-384.2488, 81.192) knots 0 0 0 1 1 1
  spline S83 degree 2 poles (-384.2488, 81.192) (-384.4016, 81.192) (-384.5458, 81.0364) (-384.5458, 80.9062) knots 0 0 0 1 2 2 2
  line L92 (-384.5458, 80.9062) -> (-384.5458, 80.7563)
  line L93 (-384.5458, 80.7563) -> (-384.0422, 80.7563)
  line L94 (-384.0422, 80.7563) -> (-384.0422, 80.1282)
  line L95 (-384.0422, 80.1282) -> (-384.5458, 80.1282)
  line L96 (-384.5458, 80.1282) -> (-384.5458, 78.5777)
  line L97 (-384.5458, 78.5777) -> (-385.4512, 78.5777)
  line L98 (-385.4512, 78.5777) -> (-385.4512, 80.1282)
  line L99 (-385.4512, 80.1282) -> (-385.8162, 80.1282)
  line L100 (-385.8162, 80.1282) -> (-385.8162, 80.7563)
  line L101 (-385.8162, 80.7563) -> (-385.4512, 80.7563)
  line L102 (-385.4512, 80.7563) -> (-385.4512, 80.9572)
  spline S84 degree 2 poles (-385.4512, 80.9572) (-385.4512, 81.2231) (-385.2051, 81.6277) (-384.7354, 81.8541) (-384.3987, 81.8541) knots 0 0 0 1 2 3 3 3
  spline S85 degree 2 poles (-384.3987, 81.8541) (-384.1554, 81.8541) (-383.9885, 81.806) knots 0 0 0 1 1 1
  line L103 (-383.9885, 81.806) -> (-383.9885, 81.1439)
  line L104 (-382.5795, 78.5777) -> (-382.5795, 78.9087)
  line L105 (-382.5795, 78.9087) -> (-382.588, 78.9087)
  spline S86 degree 2 poles (-382.588, 78.9087) (-382.8058, 78.524) (-383.2529, 78.524) knots 0 0 0 1 1 1
  spline S87 degree 2 poles (-383.2529, 78.524) (-383.5612, 78.524) (-383.9093, 78.8889) (-383.9093, 79.1973) knots 0 0 0 1 2 2 2
  spline S88 degree 2 poles (-383.9093, 79.1973) (-383.9093, 79.8396) (-383.1199, 79.9414) knots 0 0 0 1 1 1
  line L106 (-383.1199, 79.9414) -> (-382.5795, 80.0122)
  spline S89 degree 2 poles (-382.5795, 80.0122) (-382.5795, 80.1197) (-382.7719, 80.2555) (-382.9331, 80.2555) knots 0 0 0 1 2 2 2
  spline S90 degree 2 poles (-382.9331, 80.2555) (-383.2981, 80.2555) (-383.7055, 80.0461) knots 0 0 0 1 1 1
  line L107 (-383.7055, 80.0461) -> (-383.7055, 80.6346)
  spline S91 degree 2 poles (-383.7055, 80.6346) (-383.5301, 80.711) (-382.9954, 80.81) (-382.8058, 80.81) knots 0 0 0 1 2 2 2
  spline S92 degree 2 poles (-382.8058, 80.81) (-382.2513, 80.81) (-381.7505, 80.3347) (-381.7505, 79.7802) knots 0 0 0 1 2 2 2
  line L108 (-381.7505, 79.7802) -> (-381.7505, 78.5777)
  line L109 (-381.7505, 78.5777) -> (-382.5795, 78.5777)
  spline S93 degree 2 poles (-383.117, 79.319) (-383.117, 79.2313) (-383.0039, 79.1153) (-382.8992, 79.1153) knots 0 0 0 1 2 2 2
  spline S94 degree 2 poles (-382.8992, 79.1153) (-382.7577, 79.1153) (-382.5795, 79.3275) (-382.5795, 79.4944) knots 0 0 0 1 2 2 2
  line L110 (-382.5795, 79.4944) -> (-382.5795, 79.5765)
  line L111 (-382.5795, 79.5765) -> (-382.8879, 79.534)
  spline S95 degree 2 poles (-382.8879, 79.534) (-383.117, 79.4944) (-383.117, 79.319) knots 0 0 0 1 1 1
  line L112 (-379.9312, 78.5777) -> (-379.9312, 79.766)
  spline S96 degree 2 poles (-379.9312, 79.766) (-379.9312, 79.9697) (-380.0529, 80.1452) (-380.1887, 80.1452) knots 0 0 0 1 2 2 2
  spline S97 degree 2 poles (-380.1887, 80.1452) (-380.3047, 80.1452) (-380.4377, 79.9612) (-380.4377, 79.8198) knots 0 0 0 1 2 2 2
  line L113 (-380.4377, 79.8198) -> (-380.4377, 78.5777)
  line L114 (-380.4377, 78.5777) -> (-381.3431, 78.5777)
  line L115 (-381.3431, 78.5777) -> (-381.3431, 80.7563)
  line L116 (-381.3431, 80.7563) -> (-380.4377, 80.7563)
  line L117 (-380.4377, 80.7563) -> (-380.4377, 80.4168)
  line L118 (-380.4377, 80.4168) -> (-380.4292, 80.4168)
  spline S98 degree 2 poles (-380.4292, 80.4168) (-380.3217, 80.6035) (-379.9539, 80.81) (-379.7388, 80.81) knots 0 0 0 1 2 2 2
  spline S99 degree 2 poles (-379.7388, 80.81) (-379.0259, 80.81) (-379.0259, 79.9075) knots 0 0 0 1 1 1
  line L119 (-379.0259, 79.9075) -> (-379.0259, 78.5777)
  line L120 (-379.0259, 78.5777) -> (-379.9312, 78.5777)
  spline S100 degree 2 poles (-376.1937, 79.7066) (-376.1937, 79.1549) (-376.8586, 78.524) (-377.4556, 78.524) knots 0 0 0 1 2 2 2
  spline S101 degree 2 poles (-377.4556, 78.524) (-378.0497, 78.524) (-378.7118, 79.1379) (-378.7118, 79.6811) knots 0 0 0 1 2 2 2
  spline S102 degree 2 poles (-378.7118, 79.6811) (-378.7118, 80.0263) (-378.4006, 80.5384) (-377.8262, 80.81) (-377.4528, 80.81) knots 0 0 0 1 2 3 3 3
  spline S103 degree 2 poles (-377.4528, 80.81) (-377.0651, 80.81) (-376.4965, 80.5243) (-376.1937, 80.0178) (-376.1937, 79.7066) knots 0 0 0 1 2 3 3 3
  spline S104 degree 2 poles (-377.1132, 79.701) (-377.1132, 80.1452) (-377.4528, 80.1452) knots 0 0 0 1 1 1
  spline S105 degree 2 poles (-377.4528, 80.1452) (-377.7923, 80.1452) (-377.7923, 79.6811) knots 0 0 0 1 1 1
  spline S106 degree 2 poles (-377.7923, 79.6811) (-377.7923, 79.1888) (-377.4471, 79.1888) knots 0 0 0 1 1 1
  spline S107 degree 2 poles (-377.4471, 79.1888) (-377.1132, 79.1888) (-377.1132, 79.701) knots 0 0 0 1 1 1
  line L121 (-374.5612, 78.5777) -> (-374.5612, 81.6277)
  line L122 (-374.5612, 81.6277) -> (-372.6627, 81.6277)
  line L123 (-372.6627, 81.6277) -> (-372.6627, 80.9091)
  line L124 (-372.6627, 80.9091) -> (-373.6417, 80.9091)
  line L125 (-373.6417, 80.9091) -> (-373.6417, 80.4649)
  line L126 (-373.6417, 80.4649) -> (-372.7221, 80.4649)
  line L127 (-372.7221, 80.4649) -> (-372.7221, 79.7462)
  line L128 (-372.7221, 79.7462) -> (-373.6417, 79.7462)
  line L129 (-373.6417, 79.7462) -> (-373.6417, 79.2964)
  line L130 (-373.6417, 79.2964) -> (-372.592, 79.2964)
  line L131 (-372.592, 79.2964) -> (-372.592, 78.5777)
  line L132 (-372.592, 78.5777) -> (-374.5612, 78.5777)
  line L133 (-369.4147, 78.5777) -> (-369.4147, 79.8339)
  spline S108 degree 2 poles (-369.4147, 79.8339) (-369.4147, 79.9895) (-369.5279, 80.1452) (-369.6552, 80.1452) knots 0 0 0 1 2 2 2
  spline S109 degree 2 poles (-369.6552, 80.1452) (-369.7797, 80.1452) (-369.9211, 79.9556) (-369.9211, 79.7887) knots 0 0 0 1 2 2 2
  line L134 (-369.9211, 79.7887) -> (-369.9211, 78.5777)
  line L135 (-369.9211, 78.5777) -> (-370.8265, 78.5777)
  line L136 (-370.8265, 78.5777) -> (-370.8265, 79.8113)
  spline S110 degree 2 poles (-370.8265, 79.8113) (-370.8265, 80.1452) (-371.0529, 80.1452) knots 0 0 0 1 1 1
  spline S111 degree 2 poles (-371.0529, 80.1452) (-371.1915, 80.1452) (-371.333, 79.9528) (-371.333, 79.7717) knots 0 0 0 1 2 2 2
  line L137 (-371.333, 79.7717) -> (-371.333, 78.5777)
  line L138 (-371.333, 78.5777) -> (-372.2383, 78.5777)
  line L139 (-372.2383, 78.5777) -> (-372.2383, 80.7563)
  line L140 (-372.2383, 80.7563) -> (-371.333, 80.7563)
  line L141 (-371.333, 80.7563) -> (-371.333, 80.4111)
  line L142 (-371.333, 80.4111) -> (-371.3245, 80.4111)
  spline S112 degree 2 poles (-371.3245, 80.4111) (-371.2735, 80.5016) (-371.05, 80.694) (-370.7699, 80.81) (-370.6058, 80.81) knots 0 0 0 1 2 3 3 3
  spline S113 degree 2 poles (-370.6058, 80.81) (-370.3738, 80.81) (-370.0569, 80.6261) (-369.9522, 80.4281) knots 0 0 0 1 2 2 2
  spline S114 degree 2 poles (-369.9522, 80.4281) (-369.8362, 80.612) (-369.4515, 80.81) (-369.2195, 80.81) knots 0 0 0 1 2 2 2
  spline S115 degree 2 poles (-369.2195, 80.81) (-368.8743, 80.81) (-368.5093, 80.363) (-368.5093, 79.9414) knots 0 0 0 1 2 2 2
  line L143 (-368.5093, 79.9414) -> (-368.5093, 78.5777)
  line L144 (-368.5093, 78.5777) -> (-369.4147, 78.5777)
  line L145 (-366.8909, 78.5777) -> (-366.8909, 78.9087)
  line L146 (-366.8909, 78.9087) -> (-366.8994, 78.9087)
  spline S116 degree 2 poles (-366.8994, 78.9087) (-367.1173, 78.524) (-367.5643, 78.524) knots 0 0 0 1 1 1
  spline S117 degree 2 poles (-367.5643, 78.524) (-367.8727, 78.524) (-368.2207, 78.8889) (-368.2207, 79.1973) knots 0 0 0 1 2 2 2
  spline S118 degree 2 poles (-368.2207, 79.1973) (-368.2207, 79.8396) (-367.4313, 79.9414) knots 0 0 0 1 1 1
  line L147 (-367.4313, 79.9414) -> (-366.8909, 80.0122)
  spline S119 degree 2 poles (-366.8909, 80.0122) (-366.8909, 80.1197) (-367.0833, 80.2555) (-367.2446, 80.2555) knots 0 0 0 1 2 2 2
  spline S120 degree 2 poles (-367.2446, 80.2555) (-367.6096, 80.2555) (-368.017, 80.0461) knots 0 0 0 1 1 1
  line L148 (-368.017, 80.0461) -> (-368.017, 80.6346)
  spline S121 degree 2 poles (-368.017, 80.6346) (-367.8416, 80.711) (-367.3068, 80.81) (-367.1173, 80.81) knots 0 0 0 1 2 2 2
  spline S122 degree 2 poles (-367.1173, 80.81) (-366.5627, 80.81) (-366.0619, 80.3347) (-366.0619, 79.7802) knots 0 0 0 1 2 2 2
  line L149 (-366.0619, 79.7802) -> (-366.0619, 78.5777)
  line L150 (-366.0619, 78.5777) -> (-366.8909, 78.5777)
  spline S123 degree 2 poles (-367.4285, 79.319) (-367.4285, 79.2313) (-367.3153, 79.1153) (-367.2106, 79.1153) knots 0 0 0 1 2 2 2
  spline S124 degree 2 poles (-367.2106, 79.1153) (-367.0692, 79.1153) (-366.8909, 79.3275) (-366.8909, 79.4944) knots 0 0 0 1 2 2 2
  line L151 (-366.8909, 79.4944) -> (-366.8909, 79.5765)
  line L152 (-366.8909, 79.5765) -> (-367.1993, 79.534)
  spline S125 degree 2 poles (-367.1993, 79.534) (-367.4285, 79.4944) (-367.4285, 79.319) knots 0 0 0 1 1 1
  line L153 (-364.2427, 78.5777) -> (-364.2427, 79.766)
  spline S126 degree 2 poles (-364.2427, 79.766) (-364.2427, 79.9697) (-364.3644, 80.1452) (-364.5002, 80.1452) knots 0 0 0 1 2 2 2
  spline S127 degree 2 poles (-364.5002, 80.1452) (-364.6162, 80.1452) (-364.7491, 79.9612) (-364.7491, 79.8198) knots 0 0 0 1 2 2 2
  line L154 (-364.7491, 79.8198) -> (-364.7491, 78.5777)
  line L155 (-364.7491, 78.5777) -> (-365.6545, 78.5777)
  line L156 (-365.6545, 78.5777) -> (-365.6545, 80.7563)
  line L157 (-365.6545, 80.7563) -> (-364.7491, 80.7563)
  line L158 (-364.7491, 80.7563) -> (-364.7491, 80.4168)
  line L159 (-364.7491, 80.4168) -> (-364.7407, 80.4168)
  spline S128 degree 2 poles (-364.7407, 80.4168) (-364.6331, 80.6035) (-364.2653, 80.81) (-364.0503, 80.81) knots 0 0 0 1 2 2 2
  spline S129 degree 2 poles (-364.0503, 80.81) (-363.3373, 80.81) (-363.3373, 79.9075) knots 0 0 0 1 1 1
  line L160 (-363.3373, 79.9075) -> (-363.3373, 78.5777)
  line L161 (-363.3373, 78.5777) -> (-364.2427, 78.5777)
  line L162 (-361.5407, 78.5777) -> (-361.5407, 78.9144)
  line L163 (-361.5407, 78.9144) -> (-361.5492, 78.9144)
  spline S130 degree 2 poles (-361.5492, 78.9144) (-361.6624, 78.7588) (-361.8434, 78.6145) (-362.0698, 78.524) (-362.2197, 78.524) knots 0 0 0 1 2 3 3 3
  spline S131 degree 2 poles (-362.2197, 78.524) (-362.5791, 78.524) (-362.9525, 78.988) (-362.9525, 79.4407) knots 0 0 0 1 2 2 2
  line L164 (-362.9525, 79.4407) -> (-362.9525, 80.7563)
  line L165 (-362.9525, 80.7563) -> (-362.0471, 80.7563)
  line L166 (-362.0471, 80.7563) -> (-362.0471, 79.5114)
  spline S132 degree 2 poles (-362.0471, 79.5114) (-362.0471, 79.1888) (-361.8067, 79.1888) knots 0 0 0 1 1 1
  spline S133 degree 2 poles (-361.8067, 79.1888) (-361.6737, 79.1888) (-361.5407, 79.3643) (-361.5407, 79.5227) knots 0 0 0 1 2 2 2
  line L167 (-361.5407, 79.5227) -> (-361.5407, 80.7563)
  line L168 (-361.5407, 80.7563) -> (-360.6353, 80.7563)
  line L169 (-360.6353, 80.7563) -> (-360.6353, 78.5777)
  line L170 (-360.6353, 78.5777) -> (-361.5407, 78.5777)
  spline S134 degree 2 poles (-359.4187, 79.4095) (-359.3961, 79.2681) (-359.1188, 79.1096) (-358.8925, 79.1096) knots 0 0 0 1 2 2 2
  spline S135 degree 2 poles (-358.8925, 79.1096) (-358.5756, 79.1096) (-358.2926, 79.2313) knots 0 0 0 1 1 1
  line L171 (-358.2926, 79.2313) -> (-358.2926, 78.6569)
  spline S136 degree 2 poles (-358.2926, 78.6569) (-358.6208, 78.524) (-359.0933, 78.524) knots 0 0 0 1 1 1
  spline S137 degree 2 poles (-359.0933, 78.524) (-359.662, 78.524) (-360.2958, 79.1068) (-360.2958, 79.6189) knots 0 0 0 1 2 2 2
  spline S138 degree 2 poles (-360.2958, 79.6189) (-360.2958, 79.9697) (-360.0185, 80.5045) (-359.4725, 80.81) (-359.1414, 80.81) knots 0 0 0 1 2 3 3 3
  spline S139 degree 2 poles (-359.1414, 80.81) (-358.8048, 80.81) (-358.3238, 80.5469) (-358.0748, 80.0688) (-358.0748, 79.749) knots 0 0 0 1 2 3 3 3
  line L172 (-358.0748, 79.749) -> (-358.0748, 79.4095)
  line L173 (-358.0748, 79.4095) -> (-359.4187, 79.4095)
  spline S140 degree 2 poles (-358.8755, 79.8849) (-358.8755, 80.2612) (-359.1443, 80.2612) knots 0 0 0 1 1 1
  spline S141 degree 2 poles (-359.1443, 80.2612) (-359.2574, 80.2612) (-359.4102, 80.0546) (-359.4244, 79.8849) knots 0 0 0 1 2 2 2
  line L174 (-359.4244, 79.8849) -> (-358.8755, 79.8849)
  line L175 (-357.7607, 78.5777) -> (-357.7607, 81.8031)
  line L176 (-357.7607, 81.8031) -> (-356.8554, 81.8031)
  line L177 (-356.8554, 81.8031) -> (-356.8554, 78.5777)
  line L178 (-356.8554, 78.5777) -> (-357.7607, 78.5777)
  spline S142 degree 2 poles (-355.6388, 79.4095) (-355.6161, 79.2681) (-355.3388, 79.1096) (-355.1125, 79.1096) knots 0 0 0 1 2 2 2
  spline S143 degree 2 poles (-355.1125, 79.1096) (-354.7956, 79.1096) (-354.5127, 79.2313) knots 0 0 0 1 1 1
  line L179 (-354.5127, 79.2313) -> (-354.5127, 78.6569)
  spline S144 degree 2 poles (-354.5127, 78.6569) (-354.8409, 78.524) (-355.3134, 78.524) knots 0 0 0 1 1 1
  spline S145 degree 2 poles (-355.3134, 78.524) (-355.8821, 78.524) (-356.5158, 79.1068) (-356.5158, 79.6189) knots 0 0 0 1 2 2 2
  spline S146 degree 2 poles (-356.5158, 79.6189) (-356.5158, 79.9697) (-356.2386, 80.5045) (-355.6925, 80.81) (-355.3615, 80.81) knots 0 0 0 1 2 3 3 3
  spline S147 degree 2 poles (-355.3615, 80.81) (-355.0248, 80.81) (-354.5438, 80.5469) (-354.2948, 80.0688) (-354.2948, 79.749) knots 0 0 0 1 2 3 3 3
  line L180 (-354.2948, 79.749) -> (-354.2948, 79.4095)
  line L181 (-354.2948, 79.4095) -> (-355.6388, 79.4095)
  spline S148 degree 2 poles (-355.0955, 79.8849) (-355.0955, 80.2612) (-355.3643, 80.2612) knots 0 0 0 1 1 1
  spline S149 degree 2 poles (-355.3643, 80.2612) (-355.4775, 80.2612) (-355.6303, 80.0546) (-355.6444, 79.8849) knots 0 0 0 1 2 2 2
  line L182 (-355.6444, 79.8849) -> (-355.0955, 79.8849)
  spline S150 degree 2 poles (-398.07, 73.6794) (-398.07, 73.5153) (-398.2397, 73.2239) (-398.5311, 73.057) (-398.6924, 73.057) knots 0 0 0 1 2 3 3 3